Autodesk Inventor part; units mm, degrees
(part 2 of 2)
sketch "Sketch9" plane through (8.2638, 25.5, 2.7512) normal (1, 0, 0) x (0, 1, 0)
  line L0 (15.6267, 14.1538) -> (10.0956, 14.1587)
  line L1 (10.0956, 14.1587) -> (4.8594, 14.1635)
  line L2 (4.8594, 14.1635) -> (4.088, 14.1641)
  line L3 (4.088, 14.1641) -> (2.3563, 14.1657)
  line L4 (2.3563, 14.1657) -> (-2.257, 14.1698)
  line L5 (-2.257, 14.1698) -> (-3.8539, 14.1713)
  line L6 (-3.8539, 14.1713) -> (-7.4375, 14.1745)
  line L7 (-7.4375, 14.1745) -> (-15.1699, 14.1815)
  line L8 (-15.1699, 14.1815) -> (-15.2319, 14.1815)
  line L9 (-11.6818, 3.3732) -> (-12.0761, 2.933)
  line L10 (-10.7844, 10.3488) -> (-15.1699, 14.1815)
  line L11 (-10.7844, 10.3488) -> (-13.8452, 7.5417)
  line L12 (-10.5757, 10.321) -> (-10.7844, 10.3488)
  line L13 (-10.9642, 6.6282) -> (-13.8452, 7.5417)
  line L14 (-10.9642, 6.6282) -> (-11.6818, 3.3732)
  line L15 (-9.678, -1.5748) -> (-9.9814, -1.1521)
  line L16 (-9.2499, 7.1724) -> (-10.9642, 6.6282)
  line L17 (-9.2003, 7.1521) -> (-9.2499, 7.1724)
  line L18 (-9.925, 1.4399) -> (-12.0761, 2.933)
  line L19 (-9.2499, 7.1724) -> (-10.5757, 10.321)
  line L20 (-9.925, 1.4399) -> (-9.9814, -1.1521)
  line L21 (-7.7475, 12.6014) -> (-7.4375, 14.1745)
  line L22 (-7.7475, 12.6014) -> (-10.5757, 10.321)
  line L23 (-9.2122, 4.3116) -> (-11.6818, 3.3732)
  line L24 (-9.2122, 4.3116) -> (-9.2003, 7.1521)
  line L25 (-7.2029, 7.4306) -> (-9.2003, 7.1521)
  line L26 (-7.2262, 2.5933) -> (-9.925, 1.4399)
  line L27 (-7.2262, 2.5933) -> (-9.2122, 4.3116)
  line L28 (-6.7305, 2.5195) -> (-7.2262, 2.5933)
  line L29 (-6.5189, 8.0514) -> (-7.2029, 7.4306)
  line L30 (-5.8401, -0.535) -> (-9.678, -1.5748)
  line L31 (-5.3398, 0.4698) -> (-5.8401, -0.535)
  line L32 (-5.3398, 0.4698) -> (-6.7305, 2.5195)
  line L33 (-6.3417, 9.2804) -> (-6.5189, 8.0514)
  line L34 (-6.3417, 9.2804) -> (-7.7475, 12.6014)
  line L35 (-6.352, 3.752) -> (-6.7305, 2.5195)
  line L36 (-6.352, 3.752) -> (-7.2029, 7.4306)
  line L37 (-3.3195, 0.7918) -> (-5.3398, 0.4698)
  line L38 (-3.5356, 6.7166) -> (-6.5189, 8.0514)
  line L39 (-3.5226, 6.6987) -> (-3.5356, 6.7166)
  line L40 (-3.7408, 5.385) -> (-6.352, 3.752)
  line L41 (-3.7408, 5.385) -> (-3.5226, 6.6987)
  line L42 (-3.477, 10.4478) -> (-6.3417, 9.2804)
  line L43 (-3.477, 10.4478) -> (-3.8539, 14.1713)
  line L44 (-2.1303, 1.9717) -> (-3.3195, 0.7918)
  line L45 (-2.0839, 2.4881) -> (-2.1303, 1.9717)
  line L46 (-2.7188, 9.871) -> (-3.477, 10.4478)
  line L47 (-2.0839, 2.4881) -> (-3.7408, 5.385)
  line L48 (-2.5276, 9.8784) -> (-2.7188, 9.871)
  line L49 (-2.7188, 9.871) -> (-3.5356, 6.7166)
  line L50 (-2.0106, 6.673) -> (-3.5226, 6.6987)
  line L51 (-0.9613, 9.0998) -> (-2.5276, 9.8784)
  line L52 (-1.0697, 11.6538) -> (-2.257, 14.1698)
  line L53 (-1.0697, 11.6538) -> (-2.5276, 9.8784)
  line L54 (-0.2079, 5.212) -> (-2.0106, 6.673)
  line L55 (-0.2079, 5.212) -> (-2.0839, 2.4881)
  line L56 (-0.7595, 8.4985) -> (-0.9613, 9.0998)
  line L57 (-0.7595, 8.4985) -> (-2.0106, 6.673)
  line L58 (0.1704, 5.3001) -> (-0.2079, 5.212)
  line L59 (0.0555, 11.2063) -> (-1.0697, 11.6538)
  line L60 (0.2384, 10.4521) -> (-0.9613, 9.0998)
  line L61 (0.2384, 10.4521) -> (0.0555, 11.2063)
  line L62 (2.7149, 0.8141) -> (-2.1303, 1.9717)
  line L63 (1.4518, 7.3795) -> (-0.7595, 8.4985)
  line L64 (2.868, 0.1938) -> (2.7149, 0.8141)
  line L65 (1.4518, 7.3795) -> (0.1704, 5.3001)
  line L66 (0.0555, 11.2063) -> (2.3563, 14.1657)
  line L67 (3.1852, 2.3794) -> (2.7149, 0.8141)
  line L68 (2.8096, 8.0422) -> (1.4518, 7.3795)
  line L69 (3.1602, 2.5218) -> (3.1852, 2.3794)
  line L70 (3.1602, 2.5218) -> (0.1704, 5.3001)
  line L71 (2.5801, 9.2559) -> (0.2384, 10.4521)
  line L72 (2.5801, 9.2559) -> (2.8096, 8.0422)
  line L73 (3.9123, 7.3853) -> (2.8096, 8.0422)
  line L74 (2.5801, 9.2559) -> (4.088, 14.1641)
  line L75 (4.2913, 6.4296) -> (3.9123, 7.3853)
  line L76 (4.2913, 6.4296) -> (3.1602, 2.5218)
  line L77 (6.412, 9.282) -> (3.9123, 7.3853)
  line L78 (6.4294, 9.2776) -> (6.412, 9.282)
  line L79 (6.4149, 9.2729) -> (4.8594, 14.1635)
  line L80 (6.8569, 5.534) -> (4.2913, 6.4296)
  line L81 (7.3482, 3.1538) -> (3.1852, 2.3794)
  line L82 (7.3482, 3.1538) -> (6.8569, 5.534)
  line L83 (7.7155, 0.1558) -> (2.868, 0.1938)
  line L84 (9.5528, 1.5223) -> (7.3482, 3.1538)
  line L85 (9.5528, 1.5223) -> (7.7155, 0.1558)
  line L86 (9.6495, 1.52) -> (9.5528, 1.5223)
  line L87 (7.8984, 6.4684) -> (6.8569, 5.534)
  line L88 (7.8838, 6.4638) -> (6.4149, 9.2729)
  line L89 (8.3371, 9.6656) -> (6.4297, 9.276)
  line L90 (10.1933, 12.4785) -> (10.0956, 14.1587)
  line L91 (10.1787, 12.4738) -> (8.3371, 9.6656)
  line L92 (9.4798, 6.7649) -> (7.8838, 6.4638)
  line L93 (9.6575, 7.3124) -> (9.4943, 6.7695)
  line L94 (9.6575, 7.3124) -> (8.3517, 9.6702)
  line L95 (11.2205, 3.8998) -> (9.6495, 1.52)
  line L96 (11.2224, 3.9754) -> (11.2205, 3.8998)
  line L97 (11.2079, 3.9708) -> (9.4798, 6.7649)
  line L98 (11.422, 8.6705) -> (9.6575, 7.3124)
  line L99 (11.8053, 9.7292) -> (10.1787, 12.4738)
  line L100 (11.8053, 9.7292) -> (11.4075, 8.6659)
  line L101 (13.0152, 6.2418) -> (11.2079, 3.9708)
  line L102 (13.0152, 6.2418) -> (11.4075, 8.6659)
  line L103 (13.3289, 9.642) -> (11.8199, 9.7338)
  line L104 (16.1386, 7.3478) -> (13.0297, 6.2465)
  line L105 (16.1386, 7.3478) -> (13.3289, 9.642)
  line L106 (13.3289, 9.642) -> (15.6267, 14.1538)
  point P0 (-25.5, -2.7512)
  point P1 (3.1602, 2.5218)
  point P2 (-6.352, 3.752)
  point P3 (-6.7305, 2.5195)
  point P4 (3.1852, 2.3794)
  point P5 (4.8594, 14.1635)
  point P6 (2.8096, 8.0422)
  point P7 (3.9123, 7.3853)
  point P8 (6.412, 9.282)
  constraints: 214 end point, 1 point on line
sketch "Sketch6" plane through (0, 0, 0) normal (1, 0, 0) x (0, 1, 0)
  line L0 (31.6549, 6.0594) -> (32.075, 5.6953)
  line L1 (32.075, 5.6953) -> (32.3975, 6.0674)
  line L2 (32.3975, 6.0674) -> (31.9774, 6.4315)
  line L3 (31.9774, 6.4315) -> (31.6549, 6.0594)
  line L4 (31.4402, 6.2454) -> (31.0322, 6.5991)
  line L5 (31.0322, 6.5991) -> (31.3547, 6.9712)
  line L6 (31.3547, 6.9712) -> (31.7627, 6.6176)
  line L7 (31.7627, 6.6176) -> (31.4402, 6.2454)
  line L8 (30.8068, 6.7944) -> (30.4919, 7.0673)
  line L9 (30.4919, 7.0673) -> (30.8634, 7.4959)
  line L10 (30.8634, 7.4959) -> (31.1783, 7.223)
  line L11 (31.1783, 7.223) -> (30.8068, 6.7944)
  line L12 (30.3122, 7.223) -> (29.8518, 7.6221)
  line L13 (29.8518, 7.6221) -> (30.2652, 8.099)
  line L14 (30.2652, 8.099) -> (30.7256, 7.7)
  line L15 (30.7256, 7.7) -> (30.3122, 7.223)
  line L16 (29.6591, 7.789) -> (29.2369, 8.328)
  line L17 (29.2369, 8.328) -> (29.9785, 8.9091)
  line L18 (29.9785, 8.9091) -> (30.4008, 8.3701)
  line L19 (30.4008, 8.3701) -> (29.6591, 7.789)
  line L20 (29.0128, 8.5054) -> (28.2357, 9.8579)
  line L21 (28.2357, 9.8579) -> (29.2002, 10.4121)
  line L22 (29.2002, 10.4121) -> (29.9773, 9.0596)
  line L23 (29.9773, 9.0596) -> (29.0128, 8.5054)
  line L24 (28.1313, 10.0396) -> (27.6871, 11.5769)
  line L25 (27.6871, 11.5769) -> (29.0097, 11.9591)
  line L26 (29.0097, 11.9591) -> (29.4539, 10.4217)
  line L27 (29.4539, 10.4217) -> (28.1313, 10.0396)
  line L28 (27.6048, 11.8616) -> (27.451, 13.6632)
  line L29 (27.451, 13.6632) -> (28.7507, 13.7742)
  line L30 (28.7507, 13.7742) -> (28.9045, 11.9726)
  line L31 (28.9045, 11.9726) -> (27.6048, 11.8616)
  line L32 (27.431, 13.8981) -> (27.5279, 15.4838)
  line L33 (27.5279, 15.4838) -> (29.2753, 15.3769)
  line L34 (29.2753, 15.3769) -> (29.1783, 13.7913)
  line L35 (29.1783, 13.7913) -> (27.431, 13.8981)
  line L36 (27.5433, 15.735) -> (27.7311, 16.384)
  line L37 (27.7311, 16.384) -> (29.5449, 15.8591)
  line L38 (29.5449, 15.8591) -> (29.3571, 15.21)
  line L39 (29.3571, 15.21) -> (27.5433, 15.735)
  point P0 (0, 0)
  constraints: 80 end point, 20 parallel, 12 point on line, 10 perpendicular
sketch "Sketch5" plane through (11.5, 25.5, 11.5) normal (0.5, 0.7071068, -0.5) x (-0.7071068, 0, -0.7071068)
  line L0 (6.8252, -1.4428) -> (7.8817, -1.4428)
  line L1 (7.8817, -1.4428) -> (7.8817, -0.2694)
  line L2 (7.8817, -0.2694) -> (6.8252, -0.2694)
  line L3 (6.8252, -0.2694) -> (6.8252, -1.4428)
  line L4 (7.7834, -0.0942) -> (7.8817, 1.0177)
  line L5 (7.8817, 1.0177) -> (6.8531, 1.1086)
  line L6 (6.8531, 1.1086) -> (6.7549, -0.0033)
  line L7 (6.7549, -0.0033) -> (7.7834, -0.0942)
  line L8 (7.9744, 1.3229) -> (8.1838, 2.5507)
  line L9 (8.1838, 2.5507) -> (6.9188, 2.7665)
  line L10 (6.9188, 2.7665) -> (6.7094, 1.5387)
  line L11 (6.7094, 1.5387) -> (7.9744, 1.3229)
  line L12 (8.2323, 2.835) -> (8.6796, 3.9697)
  line L13 (8.6796, 3.9697) -> (7.2053, 4.5509)
  line L14 (7.2053, 4.5509) -> (6.758, 3.4162)
  line L15 (6.758, 3.4162) -> (8.2323, 2.835)
  line L16 (8.7942, 4.2603) -> (9.2218, 4.9952)
  line L17 (9.2218, 4.9952) -> (8.0469, 5.6787)
  line L18 (8.0469, 5.6787) -> (7.6193, 4.9438)
  line L19 (7.6193, 4.9438) -> (8.7942, 4.2603)
  line L20 (9.4056, 5.3112) -> (10.1998, 6.1602)
  line L21 (10.1998, 6.1602) -> (9.3216, 6.9817)
  line L22 (9.3216, 6.9817) -> (8.5274, 6.1328)
  line L23 (8.5274, 6.1328) -> (9.4056, 5.3112)
  line L24 (10.5561, 6.3427) -> (11.3524, 6.8618)
  line L25 (11.3524, 6.8618) -> (10.667, 7.9132)
  line L26 (10.667, 7.9132) -> (9.8707, 7.3941)
  line L27 (9.8707, 7.3941) -> (10.5561, 6.3427)
  line L28 (11.6904, 7.0821) -> (12.8584, 7.6536)
  line L29 (12.8584, 7.6536) -> (12.0601, 9.2853)
  line L30 (12.0601, 9.2853) -> (10.892, 8.7138)
  line L31 (10.892, 8.7138) -> (11.6904, 7.0821)
  line L32 (13.0567, 7.7507) -> (14.3838, 8.2969)
  line L33 (14.3838, 8.2969) -> (13.7539, 9.8271)
  line L34 (13.7539, 9.8271) -> (12.4269, 9.2809)
  line L35 (12.4269, 9.2809) -> (13.0567, 7.7507)
  line L36 (14.6205, 8.5158) -> (15.5759, 8.6325)
  line L37 (15.5759, 8.6325) -> (15.4151, 9.9488)
  line L38 (15.4151, 9.9488) -> (14.4597, 9.8321)
  line L39 (14.4597, 9.8321) -> (14.6205, 8.5158)
  point P0 (16.2635, -18.0312)
  constraints: 80 end point, 20 parallel, 10 perpendicular, 6 point on line, 1 horizontal
body "Solid1"
